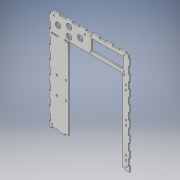
# Autodesk Inventor part: 10 voor plaat
Saved by Autodesk Inventor 2019 (Build 230136000, 136)
## iProperties
Created: 2021-01-22
Part Number: 10 voor plaat
Material: Generic
Document SubType Name: Sheet Metal
Designer: Stefan
Density: 1 g/cm^3
Sheet Metal Rule: Default_mm
Appearance: Default
Author: Stefan
Autodesk Inventor part; units mm, degrees
ref_plane "YZ Plane" through (0, 0, 0) normal (1, 0, 0) x (0, 1, 0)
ref_plane "XZ Plane" through (0, 0, 0) normal (0, 1, 0) x (-1, 0, 0)
ref_plane "XY Plane" through (0, 0, 0) normal (0, 0, 1) x (1, 0, 0)
sketch "Sketch1" plane through (0, 0, 0) normal (0, 0, 1) x (1, 0, 0)
  line L0 (-90.5, -90.5) -> (90.5, -90.5)
  line L1 (90.5, -90.5) -> (90.5, 90.5)
  line L2 (90.5, 90.5) -> (-90.5, 90.5)
  line L3 (-90.5, 90.5) -> (-90.5, -90.5)
  line L4 (-90.5, -90.5) -> (90.5, 90.5) construction
  line L5 (90.5, -90.5) -> (-90.5, 90.5) construction
  point P0 (0, 0)
  dimension "d0" = 181
  dimension "d1" = 181
  constraints: 12 end point, 2 midpoint, 2 parallel, 1 horizontal, 1 perpendicular
  measures "d0" distance of L2.end L1.end
  measures "d1" distance of L1.end L0.end
extrude "Extrusion1" add sketch "Sketch1" along normal blind 3
sketch "Sketch2" plane through (0, 0, 3) normal (0, 0, 1) x (1, 0, 0)
  line L0 (90.5, 90.5) -> (-90.5, 90.5) projected
  line L1 (-90.5, 90.5) -> (-85, 90.5)
  line L2 (-85, 90.5) -> (-85, 93.5)
  line L3 (-85, 93.5) -> (-90.5, 93.5)
  line L4 (-90.5, 93.5) -> (-90.5, 90.5)
  line L5 (80, 90.5) -> (85.5, 90.5)
  line L6 (85.5, 90.5) -> (85.5, 93.5)
  line L7 (85.5, 93.5) -> (80, 93.5)
  line L8 (80, 93.5) -> (80, 90.5)
  line L9 (-90.5, -93.5) -> (-85, -93.5)
  line L10 (-85, -93.5) -> (-85, -90.5)
  line L11 (-85, -90.5) -> (-90.5, -90.5)
  line L12 (-90.5, -90.5) -> (-90.5, -93.5)
  line L13 (80, -93.5) -> (85.5, -93.5)
  line L14 (85.5, -93.5) -> (85.5, -90.5)
  line L15 (85.5, -90.5) -> (80, -90.5)
  line L16 (80, -90.5) -> (80, -93.5)
  line L17 (-70, 90.5) -> (-55, 90.5)
  line L18 (-55, 90.5) -> (-55, 93.5)
  line L19 (-55, 93.5) -> (-70, 93.5)
  line L20 (-70, 93.5) -> (-70, 90.5)
  line L21 (-25, 90.5) -> (-25, 93.5)
  line L22 (-40, 90.5) -> (-25, 90.5)
  line L23 (-25, 93.5) -> (-40, 93.5)
  line L24 (-40, 93.5) -> (-40, 90.5)
  line L25 (5, 90.5) -> (5, 93.5)
  line L26 (-10, 90.5) -> (5, 90.5)
  line L27 (5, 93.5) -> (-10, 93.5)
  line L28 (-10, 93.5) -> (-10, 90.5)
  line L29 (35, 90.5) -> (35, 93.5)
  line L30 (20, 90.5) -> (35, 90.5)
  line L31 (35, 93.5) -> (20, 93.5)
  line L32 (20, 93.5) -> (20, 90.5)
  line L33 (65, 90.5) -> (65, 93.5)
  line L34 (50, 90.5) -> (65, 90.5)
  line L35 (65, 93.5) -> (50, 93.5)
  line L36 (50, 93.5) -> (50, 90.5)
  line L37 (-55, -93.5) -> (-55, -90.5)
  line L38 (-70, -93.5) -> (-55, -93.5)
  line L39 (-55, -90.5) -> (-70, -90.5)
  line L40 (-70, -90.5) -> (-70, -93.5)
  line L41 (-25, -93.5) -> (-25, -90.5)
  line L42 (-40, -93.5) -> (-25, -93.5)
  line L43 (-25, -90.5) -> (-40, -90.5)
  line L44 (-40, -90.5) -> (-40, -93.5)
  line L45 (5, -93.5) -> (5, -90.5)
  line L46 (-10, -93.5) -> (5, -93.5)
  line L47 (5, -90.5) -> (-10, -90.5)
  line L48 (-10, -90.5) -> (-10, -93.5)
  line L49 (35, -93.5) -> (35, -90.5)
  line L50 (20, -93.5) -> (35, -93.5)
  line L51 (35, -90.5) -> (20, -90.5)
  line L52 (20, -90.5) -> (20, -93.5)
  line L53 (65, -93.5) -> (65, -90.5)
  line L54 (50, -93.5) -> (65, -93.5)
  line L55 (65, -90.5) -> (50, -90.5)
  line L56 (50, -90.5) -> (50, -93.5)
  point P0 (0, 0)
  dimension "d4" = 5.5
  dimension "d5" = 3
  dimension "d8" = 170.5
  dimension "d11" = 184
  dimension "d14" = 15
  dimension "d15" = 3
  dimension "d16" = 15
  dimension "d19" = 30
  dimension "d22" = 184
  constraints: 112 end point, 4 horizontal, 4 parallel, 3 collinear, 2 perpendicular, 2 vertical, 1 point on line, 93 other
  measures "d4" distance of L3.end L2.end
  measures "d5" distance of L2.end L1.end
  measures "d8" distance of L2.end L6.end
  measures "d11" distance of L2.end L10.end
  measures "d14" distance of L19.end L18.end
  measures "d15" distance of L18.end L17.end
  measures "d16" distance between parallel lines of L20 L2
  measures "d19" distance of L17.end L21.start
  measures "d22" distance of L17.end L37.start
extrude "Extrusion2" add sketch "Sketch2" against normal blind 3
sketch "Sketch3" plane through (0, 0, 3) normal (0, 0, 1) x (1, 0, 0)
  line L0 (-90.5, 93.5) -> (-90.5, -93.5) projected
  line L1 (-90.5, 82.5) -> (-87.5, 82.5)
  line L2 (-87.5, 82.5) -> (-87.5, 67.5)
  line L3 (-87.5, 67.5) -> (-90.5, 67.5)
  line L4 (-90.5, 67.5) -> (-90.5, 82.5)
  line L5 (-85, 93.5) -> (-90.5, 93.5) projected
  line L6 (-90.5, 52.5) -> (-87.5, 52.5)
  line L7 (-87.5, 52.5) -> (-87.5, 37.5)
  line L8 (-87.5, 37.5) -> (-90.5, 37.5)
  line L9 (-90.5, 37.5) -> (-90.5, 52.5)
  line L10 (-90.5, 22.5) -> (-87.5, 22.5)
  line L11 (-87.5, 22.5) -> (-87.5, 7.5)
  line L12 (-87.5, 7.5) -> (-90.5, 7.5)
  line L13 (-90.5, 7.5) -> (-90.5, 22.5)
  line L14 (-90.5, -7.5) -> (-87.5, -7.5)
  line L15 (-87.5, -7.5) -> (-87.5, -22.5)
  line L16 (-87.5, -22.5) -> (-90.5, -22.5)
  line L17 (-90.5, -22.5) -> (-90.5, -7.5)
  line L18 (-90.5, -37.5) -> (-87.5, -37.5)
  line L19 (-87.5, -37.5) -> (-87.5, -52.5)
  line L20 (-87.5, -52.5) -> (-90.5, -52.5)
  line L21 (-90.5, -52.5) -> (-90.5, -37.5)
  line L22 (-90.5, -67.5) -> (-87.5, -67.5)
  line L23 (-87.5, -67.5) -> (-87.5, -82.5)
  line L24 (-87.5, -82.5) -> (-90.5, -82.5)
  line L25 (-90.5, -82.5) -> (-90.5, -67.5)
  line L26 (87.5, 82.5) -> (90.5, 82.5)
  line L27 (90.5, 82.5) -> (90.5, 67.5)
  line L28 (90.5, 67.5) -> (87.5, 67.5)
  line L29 (87.5, 67.5) -> (87.5, 82.5)
  line L30 (87.5, 52.5) -> (90.5, 52.5)
  line L31 (90.5, 52.5) -> (90.5, 37.5)
  line L32 (90.5, 37.5) -> (87.5, 37.5)
  line L33 (87.5, 37.5) -> (87.5, 52.5)
  line L34 (87.5, 22.5) -> (90.5, 22.5)
  line L35 (90.5, 22.5) -> (90.5, 7.5)
  line L36 (90.5, 7.5) -> (87.5, 7.5)
  line L37 (87.5, 7.5) -> (87.5, 22.5)
  line L38 (87.5, -7.5) -> (90.5, -7.5)
  line L39 (90.5, -7.5) -> (90.5, -22.5)
  line L40 (90.5, -22.5) -> (87.5, -22.5)
  line L41 (87.5, -22.5) -> (87.5, -7.5)
  line L42 (87.5, -37.5) -> (90.5, -37.5)
  line L43 (90.5, -37.5) -> (90.5, -52.5)
  line L44 (90.5, -52.5) -> (87.5, -52.5)
  line L45 (87.5, -52.5) -> (87.5, -37.5)
  line L46 (87.5, -67.5) -> (90.5, -67.5)
  line L47 (90.5, -67.5) -> (90.5, -82.5)
  line L48 (90.5, -82.5) -> (87.5, -82.5)
  line L49 (87.5, -82.5) -> (87.5, -67.5)
  point P0 (0, 0)
  dimension "d27" = 3
  dimension "d28" = 15
  dimension "d29" = 11
  dimension "d32" = 30
  dimension "d35" = 178
  constraints: 96 end point, 2 horizontal, 2 parallel, 1 perpendicular, 1 point on line, 1 vertical, 88 other
  measures "d27" distance of L2.end L3.end
  measures "d28" distance of L1.end L2.end
  measures "d29" distance between parallel lines of L5 L1
  measures "d32" distance of L1.start L6.start
  measures "d35" distance of L1.start L26.start
extrude "Extrusion3" cut sketch "Sketch3" against normal blind 3
sketch "Sketch4" plane through (0, 0, 3) normal (0, 0, 1) x (1, 0, 0)
  line L0 (80, 93.5) -> (85.5, 93.5) projected
  line L1 (90.5, 90.5) -> (85.5, 90.5) projected
  line L2 (85.5, 93.5) -> (90.5, 93.5)
  line L3 (90.5, 93.5) -> (90.5, 90.5)
  line L4 (90.5, 90.5) -> (85.5, 90.5)
  line L5 (85.5, 90.5) -> (85.5, 93.5)
  line L6 (85.5, -90.5) -> (90.5, -90.5) projected
  line L7 (85.5, -90.5) -> (90.5, -90.5)
  line L8 (90.5, -90.5) -> (90.5, -93.5)
  line L9 (90.5, -93.5) -> (85.5, -93.5)
  line L10 (85.5, -93.5) -> (85.5, -90.5)
  point P0 (0, 0)
  dimension "d40" = 184
  constraints: 16 end point, 4 parallel, 2 horizontal, 2 perpendicular, 1 point on line
  measures "d40" distance between parallel lines of L1 L9
extrude "Extrusion4" add sketch "Sketch4" against normal blind 3
sketch "Sketch5" plane through (0, 0, 0) normal (0, 0, -1) x (-1, 0, 0)
  line L0 (-75, 93.5) -> (47.5, 93.5)
  line L1 (47.5, 93.5) -> (47.5, -93.5)
  line L2 (47.5, -93.5) -> (-75, -93.5)
  line L3 (-75, -93.5) -> (-75, 93.5)
  line L4 (-90.5, 22.5) -> (-90.5, 37.5) projected
  line L5 (90.5, 22.5) -> (90.5, 37.5) projected
  point P0 (0, 0)
  dimension "d43" = 187
  dimension "d44" = 15.5
  dimension "d45" = 43
  dimension "d46" = 93.5
  constraints: 8 end point, 2 parallel, 1 horizontal, 1 perpendicular
  measures "d43" distance of L0.end L1.end
  measures "d44" distance between parallel lines of L3 L4
  measures "d45" distance between parallel lines of L5 L1
  measures "d46" distance from line of point (0, 0) L0
extrude "Extrusion5" cut sketch "Sketch5" against normal blind 10
sketch "Sketch6" plane through (0, 0, 0) normal (0, 0, -1) x (-1, 0, 0)
  line L0 (-87.5, 82.5) -> (-90.5, 82.5)
  circle A0 centre (-83, 73.5) radius 2
  circle A1 centre (-83, 63.5) radius 2
  line L1 (-87.5, 82.5) -> (-87.5, 67.5)
  line L2 (-80, 93.5) -> (-90.5, 93.5)
  circle A2 centre (-83, -73.5) radius 2
  circle A3 centre (-83, -63.5) radius 2
  line L3 (-87.5, -67.5) -> (-87.5, -82.5)
  line L4 (-90.5, -93.5) -> (-80, -93.5)
  circle A4 centre (-83, 5) radius 2
  circle A5 centre (-83, -5) radius 2
  line L5 (-87.5, 22.5) -> (-87.5, 7.5)
  line L6 (-90.5, -7.5) -> (-87.5, -7.5)
  line L7 (52.75, -25) -> (72.95, -25) construction
  line L8 (72.95, -25) -> (72.95, 15) construction
  line L9 (72.95, 15) -> (52.75, 15) construction
  line L10 (52.75, 15) -> (52.75, -25) construction
  circle A6 centre (52.75, 15) radius 2
  circle A7 centre (72.95, 15) radius 2
  circle A8 centre (72.95, -25) radius 2
  circle A9 centre (52.75, -25) radius 2
  point P0 (0, 0)
  point P1 (0, 0)
  dimension "d49" = 4
  dimension "d50" = 4
  dimension "d51" = 10
  dimension "d52" = 4.5
  dimension "d53" = 0
  dimension "d54" = 20
  dimension "d55" = 4
  dimension "d56" = 4
  dimension "d57" = 10
  dimension "d58" = 4.5
  dimension "d59" = 4.5
  dimension "d60" = 20
  dimension "d61" = 4
  dimension "d62" = 4
  dimension "d63" = 0
  dimension "d64" = 10
  dimension "d65" = 4.5
  dimension "d66" = 2.5
  dimension "d67" = 20.2
  dimension "d68" = 40
  dimension "d69" = 72.95
  dimension "d70" = 15
  dimension "d71" = 4
  dimension "d72" = 4
  dimension "d73" = 4
  dimension "d74" = 4
  dimension "d75" = 90
  dimension "d76" = 90
  dimension "d77" = 160.45
  dimension "d78" = 78.5
  dimension "d79" = 67.5
  dimension "d80" = 22.5
  dimension "d81" = 108.5
  dimension "d82" = 72.95
  dimension "d83" = 15
  dimension "d84" = 87.5
  dimension "d85" = 87.5
  dimension "d86" = 152.95
  dimension "d87" = 152.95
  dimension "d88" = 52.5
  dimension "d89" = 7.5
  dimension "d90" = 7.5
  dimension "d91" = 160.45
  dimension "d92" = 82.5
  dimension "d93" = 97.5
  dimension "d94" = 163.45
  dimension "d95" = 163.45
  dimension "d96" = 163.45
  dimension "d97" = 163.45
  constraints: 22 end point, 10 centre point, 7 parallel, 4 coincident, 1 horizontal, 1 perpendicular
  measures "d49" diameter of A0
  measures "d50" diameter of A1
  measures "d51" distance of A0.centre A1.centre
  measures "d52" distance from line of L1 A0.centre
  measures "d53" horizontal distance of A0.centre A1.centre
  measures "d54" distance from line of L2 A0.centre
  measures "d55" diameter of A2
  measures "d56" diameter of A3
  measures "d57" distance of A3.centre A2.centre
  measures "d58" distance from line of A3.centre L3
  measures "d59" distance from line of L3 A2.centre
  measures "d60" distance from line of L4 A2.centre
  measures "d61" diameter of A4
  measures "d62" diameter of A5
  measures "d63" horizontal distance of A4.centre A5.centre
  measures "d64" distance of A4.centre A5.centre
  measures "d65" distance from line of L5 A5.centre
  measures "d66" distance from line of A5.centre L6
  measures "d67" distance of L9.end L8.end
  measures "d68" distance of L8.end L7.end
  measures "d69" distance from line of point (0, 0) L8
  measures "d70" distance from line of point (0, 0) L9
  measures "d71" diameter of A6
  measures "d72" diameter of A9
  measures "d73" diameter of A8
  measures "d74" diameter of A7
  measures "d75" angle of L1 L9
  measures "d76" angle of L3 L9
  measures "d77" distance between parallel lines of L5 L8
  measures "d78" distance between parallel lines of L2 L9
  measures "d79" distance between parallel lines of L0 L9
  measures "d80" distance between parallel lines of L6 L9
  measures "d81" distance between parallel lines of L4 L9
  measures "d82" distance from line of point (0, 0) L8
  measures "d83" distance from line of point (0, 0) L9
  measures "d84" distance from line of point (0, 0) L1
  measures "d85" distance from line of point (0, 0) L3
  measures "d86" distance from line of L2.start L8
  measures "d87" distance from line of L4.end L8
  measures "d88" distance from line of L1.end L9
  measures "d89" distance from line of L5.start L9
  measures "d90" distance from line of L5.end L9
  measures "d91" distance from line of L6.end L8
  measures "d92" distance from line of L3.start L9
  measures "d93" distance from line of L3.end L9
  measures "d94" distance from line of L2.end L8
  measures "d95" distance from line of L0.end L8
  measures "d96" distance from line of L6.start L8
  measures "d97" distance from line of L4.start L8
extrude "Extrusion6" cut sketch "Sketch6" against normal blind 10
sketch "Sketch8" plane through (0, 0, 0) normal (0, 0, -1) x (-1, 0, 0)
  line L0 (-90.5, 82.5) -> (-90.5, 93.5)
  line L1 (-90.5, 93.5) -> (90.5, 93.5)
  line L2 (90.5, 93.5) -> (90.5, 133.5)
  line L3 (90.5, 133.5) -> (-90.5, 133.5)
  line L4 (-90.5, 133.5) -> (-90.5, 93.5)
  line L5 (-76.15, 101.2) -> (-4.85, 101.2)
  line L6 (-4.85, 101.2) -> (-4.85, 125.8)
  line L7 (-4.85, 125.8) -> (-76.15, 125.8)
  line L8 (-76.15, 125.8) -> (-76.15, 101.2)
  line L9 (-76.15, 101.2) -> (-4.85, 125.8) construction
  line L10 (-4.85, 101.2) -> (-76.15, 125.8) construction
  line L11 (-78.025, 98) -> (-2.975, 98) construction
  line L12 (-2.975, 98) -> (-2.975, 129) construction
  line L13 (-2.975, 129) -> (-78.025, 129) construction
  line L14 (-78.025, 129) -> (-78.025, 98) construction
  line L15 (-78.025, 98) -> (-2.975, 129) construction
  line L16 (-2.975, 98) -> (-78.025, 129) construction
  circle A0 centre (-2.975, 129) radius 1.5
  circle A1 centre (-2.975, 98) radius 1.5
  circle A2 centre (-78.025, 98) radius 1.5
  circle A3 centre (-78.025, 129) radius 1.5
  circle A4 centre (45.25, 103.75) radius 6.15
  circle A5 centre (45.25, 103.75) radius 8.25 construction
  circle A6 centre (70.25, 113.5) radius 6.15
  circle A7 centre (70.25, 113.5) radius 8.25 construction
  circle A8 centre (45.25, 123.25) radius 6.15
  circle A9 centre (45.25, 123.25) radius 8.25 construction
  circle A10 centre (20.25, 113.5) radius 6.15
  circle A11 centre (20.25, 113.5) radius 8.25 construction
  point P0 (0, 0)
  point P1 (0, 0)
  point P2 (-40.5, 113.5)
  dimension "d150" = 181
  dimension "d151" = 40
  dimension "d152" = 71.3
  dimension "d153" = 24.6
  dimension "d154" = 31
  dimension "d155" = 75.05
  dimension "d156" = 3
  dimension "d157" = 3
  dimension "d158" = 3
  dimension "d159" = 3
  dimension "d160" = 20
  dimension "d161" = 50
  dimension "d162" = 12.3
  dimension "d163" = 16.5
  dimension "d164" = 12.3
  dimension "d165" = 16.5
  dimension "d166" = 12.3
  dimension "d167" = 16.5
  dimension "d168" = 12.3
  dimension "d169" = 16.5
  dimension "d170" = 45.25
  dimension "d171" = 45.25
  dimension "d172" = 2
  dimension "d173" = 2
  dimension "d174" = 20
  dimension "d175" = 20
  dimension "d176" = 90.5
  dimension "d177" = 25
  dimension "d178" = 25
  dimension "d179" = 90
  dimension "d180" = 90.5
  dimension "d181" = 133.5
  dimension "d182" = 20.25
  dimension "d183" = 133.5
  dimension "d184" = 51
  constraints: 34 end point, 12 centre point, 8 coincident, 6 parallel, 4 midpoint, 3 horizontal, 3 perpendicular
  measures "d150" distance of L4.start L3.start
  measures "d151" distance of L3.start L1.end
  measures "d152" distance of L8.start L6.end
  measures "d153" distance of L6.end L6.start
  measures "d154" distance of L12.end L12.start
  measures "d155" distance of L12.end L14.start
  measures "d156" diameter of A0
  measures "d157" diameter of A1
  measures "d158" diameter of A2
  measures "d159" diameter of A3
  measures "d160" distance from line of L3 point (-40.5, 113.5)
  measures "d161" distance from line of point (-40.5, 113.5) L4
  measures "d162" diameter of A4
  measures "d163" diameter of A5
  measures "d164" diameter of A6
  measures "d165" diameter of A7
  measures "d166" diameter of A8
  measures "d167" diameter of A9
  measures "d168" diameter of A10
  measures "d169" diameter of A11
  measures "d170" horizontal distance of A9.centre point (0, 0)
  measures "d171" horizontal distance of A4.centre point (0, 0)
  measures "d172" distance edge to line of A9 L3
  measures "d173" distance edge to line of A5 L1
  measures "d174" distance from line of A6.centre L3
  measures "d175" distance from line of L3 A11.centre
  measures "d176" horizontal distance of L1.end point (0, 0)
  measures "d177" horizontal distance of A8.centre A11.centre
  measures "d178" horizontal distance of A9.centre A6.centre
  measures "d179" angle of L0 L3
  measures "d180" distance from line of point (0, 0) L2
  measures "d181" distance from line of point (0, 0) L3
  measures "d182" distance from line of A6.centre L2
  measures "d183" distance from line of point (0, 0) L3
  measures "d184" distance from line of L0.start L3
extrude "Extrusion8" add sketch "Sketch8" against normal blind 3
sketch "Sketch9" plane through (0, 0, 0) normal (0, 0, -1) x (-1, 0, 0)
  line L0 (8.25, 102.222) -> (14.25, 102.222)
  line L1 (15.25, 102.222) -> (15.25, 94.222)
  line L2 (15.25, 94.222) -> (7.25, 94.222)
  line L3 (7.25, 94.222) -> (7.25, 102.222)
  line L4 (7.25, 102.222) -> (15.25, 94.222) construction
  line L5 (15.25, 102.222) -> (7.25, 94.222) construction
  arc A0 (15.25, 102.222) -> (7.25, 102.222) centre (11.25, 102.222) ccw
  arc A1 (14.25, 102.222) -> (8.25, 102.222) centre (11.25, 102.222) ccw
  arc A2 (11.75, 97.356) -> (10.75, 97.356) centre (11.25, 98.222) ccw
  line L6 (10.75, 95.722) -> (11.75, 95.722)
  line L7 (10.75, 95.722) -> (11.75, 98.722) construction
  line L8 (11.75, 95.722) -> (10.75, 98.722) construction
  line L9 (10.75, 97.356) -> (10.75, 95.722)
  line L10 (11.75, 95.722) -> (11.75, 97.356)
  line L11 (55, 93.5) -> (-80, 93.5) projected
  circle A3 centre (20.25, 113.5) radius 6.15 projected
  circle A4 centre (20.25, 113.5) radius 8 construction
  point P0 (0, 0)
  dimension "d187" = 8
  dimension "d188" = 8
  dimension "d189" = 1
  dimension "d190" = 2
  dimension "d191" = 1
  dimension "d192" = 3
  dimension "d193" = 0.722
  dimension "d194" = 16
  dimension "d195" = 9
  dimension "d196" = 71.565
  dimension "d197" = 108.435
  dimension "d198" = 8.722
  dimension "d199" = 2.222
  dimension "d200" = 3.5
  dimension "d201" = 4.5
  constraints: 22 end point, 6 point on circle, 4 centre point, 3 parallel, 2 coincident, 2 horizontal, 2 midpoint, 2 perpendicular, 2 tangent
  measures "d187" distance of L1.end L2.end
  measures "d188" distance of L1.start L1.end
  measures "d189" radial gap between concentric circles of A0 A1
  measures "d190" diameter of A2
  measures "d191" distance of L8.end L7.end
  measures "d192" distance of L7.end L6.end
  measures "d193" distance between parallel lines of L11 L2
  measures "d194" diameter of A4
  measures "d195" horizontal distance of A4.centre point (11.25, 98.222)
  measures "d196" angle of L8 L11
  measures "d197" angle of L7 L11
  measures "d198" distance between parallel lines of L0 L11
  measures "d199" distance between parallel lines of L6 L11
  measures "d200" distance between parallel lines of L10 L1
  measures "d201" distance between parallel lines of L9 L1
extrude "Extrusion9" add sketch "Sketch9" along normal blind 0.2 contours L1 L2 L3 A0
sketch "Sketch10" plane through (0, 0, 0) normal (0, 0, -1) x (-1, 0, 0)
  circle A0 centre (45.25, 123.25) radius 6.15 construction
  circle A1 centre (45.25, 103.75) radius 6.15 construction
  circle A2 centre (45.25, 103.75) radius 8 construction
  circle A3 centre (70.25, 113.5) radius 6.15 construction
  circle A4 centre (70.25, 113.5) radius 8 construction
  line L0 (32.25, 123.25) -> (32.25, 131.6682) construction
  line L1 (32.25, 103.75) -> (32.25, 95.75) construction
  line L2 (32.25, 131.6682) -> (35.8952, 125.3545)
  line L3 (35.8952, 125.3545) -> (28.6048, 125.3545)
  line L4 (28.6048, 125.3545) -> (32.25, 131.6682)
  line L5 (32.25, 95.75) -> (28.7859, 101.75)
  line L6 (28.7859, 101.75) -> (35.7141, 101.75)
  line L7 (35.7141, 101.75) -> (32.25, 95.75)
  line L8 (70.25, 113.5) -> (58.25, 113.5) construction
  line L9 (53.0987, 113.4997) -> (54.5129, 114.9139)
  line L10 (54.5129, 114.9139) -> (55.9271, 113.4997)
  line L11 (53.0987, 113.4997) -> (55.0987, 113.4997) construction
  line L12 (55.9271, 113.4997) -> (60.1698, 117.7424)
  line L13 (60.1698, 117.7424) -> (61.584, 116.3281)
  line L14 (61.584, 116.3281) -> (55.9271, 110.6713)
  line L15 (53.0987, 113.4997) -> (55.9271, 110.6713)
  line L16 (32.25, 123.25) -> (45.25, 123.25) construction
  line L17 (32.25, 103.75) -> (45.25, 103.75) construction
  circle A5 centre (45.25, 123.25) radius 8 construction
  point P0 (0, 0)
  point P1 (32.25, 127.4591)
  point P2 (32.25, 99.75)
  dimension "d205" = 16
  dimension "d206" = 16
  dimension "d207" = 13
  dimension "d208" = 13
  dimension "d211" = 12
  dimension "d212" = 2
  dimension "d213" = 45
  dimension "d217" = 6
  dimension "d218" = 2
  dimension "d219" = 4.128
  dimension "d223" = 0.0003
  dimension "d224" = 4
  dimension "d259" = 16
  dimension "d260" = 11.8545
  dimension "d261" = 11.75
  constraints: 36 end point, 6 parallel, 4 horizontal, 3 centre point, 3 coincident, 2 midpoint, 1 equal length, 1 perpendicular, 14 other
  measures "d205" diameter of A2
  measures "d206" diameter of A4
  measures "d207" distance of L16.end L0.start
  measures "d208" distance of L17.end L1.start
  measures "d211" distance of L8.start L8.end
  measures "d212" distance of L9.start L9.end
  measures "d213" angle of L11 L9
  measures "d217" distance between parallel lines of L13 L10
  measures "d218" distance between parallel lines of L14 L12
  measures "d219" distance from line of L8.start L13
  measures "d223" distance between parallel lines of L8 L11
  measures "d224" distance between parallel lines of L14 L9
  measures "d259" diameter of A5
  measures "d260" distance between parallel lines of L3 L8
  measures "d261" distance between parallel lines of L8 L6
extrude "Extrusion10" add sketch "Sketch10" along normal blind 0.2
fillet "Fillet1" radius 0.75 5 edges at (-61.584, 116.3281, -0.1) (-60.1698, 117.7424, -0.1) (-54.5129, 114.9139, -0.1) (-53.0987, 113.4997, -0.1) (-55.9271, 110.6713, -0.1)
sketch "Sketch11" plane through (0, 0, 0) normal (0, 0, -1) x (-1, 0, 0)
  line L0 (-90.5, 82.5) -> (-90.5, 97.5) construction
  line L1 (-90.5, 97.5) -> (-87.5, 97.5)
  line L2 (-87.5, 97.5) -> (-87.5, 112.5)
  line L3 (-87.5, 112.5) -> (-90.5, 112.5)
  line L4 (-90.5, 112.5) -> (-90.5, 97.5)
  line L5 (-90.5, 112.5) -> (-90.5, 127.5) construction
  line L6 (-90.5, 127.5) -> (-87.5, 127.5)
  line L7 (-87.5, 127.5) -> (-87.5, 133.5)
  line L8 (-90.5, 133.5) -> (-90.5, 127.5)
  line L9 (90.5, 82.5) -> (87.5, 82.5) construction
  line L10 (90.5, 82.5) -> (90.5, 97.5) construction
  line L11 (90.5, 97.5) -> (87.5, 97.5)
  line L12 (87.5, 97.5) -> (87.5, 112.5)
  line L13 (87.5, 112.5) -> (90.5, 112.5)
  line L14 (90.5, 112.5) -> (90.5, 97.5)
  line L15 (90.5, 112.5) -> (90.5, 127.5) construction
  line L16 (90.5, 127.5) -> (87.5, 127.5)
  line L17 (87.5, 127.5) -> (87.5, 133.5)
  line L18 (87.5, 133.5) -> (90.5, 133.5)
  line L19 (90.5, 133.5) -> (90.5, 127.5)
  line L20 (-90.5, 133.5) -> (90.5, 133.5) construction
  line L21 (-90.5, 133.5) -> (-87.5, 133.5)
  point P0 (0, 0)
  dimension "d225" = 15
  dimension "d226" = 3
  dimension "d227" = 15
  dimension "d228" = 15
  dimension "d229" = 15
  dimension "d230" = 3
  dimension "d231" = 15
  dimension "d232" = 15
  dimension "d233" = 90
  dimension "d234" = 90
  dimension "d235" = 3
  dimension "d236" = 178
  constraints: 40 end point, 7 parallel, 4 horizontal, 4 perpendicular, 1 collinear
  measures "d225" distance of L0.start L0.end
  measures "d226" distance of L3.end L2.end
  measures "d227" distance of L2.end L1.end
  measures "d228" distance of L3.end L5.end
  measures "d229" distance of L9.start L10.end
  measures "d230" distance of L12.end L13.end
  measures "d231" distance of L11.end L12.end
  measures "d232" distance of L13.end L15.end
  measures "d233" angle of L9 L15
  measures "d234" angle of L9 L5
  measures "d235" distance between parallel lines of L17 L19
  measures "d236" distance between parallel lines of L19 L7
extrude "Extrusion11" cut sketch "Sketch11" against normal blind 3
sketch "Sketch12" plane through (0, 0, 0) normal (0, 0, -1) x (-1, 0, 0)
  line L0 (-87.5, 133.5) -> (87.5, 133.5) projected
  line L1 (-82.5, 133.5) -> (-67.5, 133.5)
  line L2 (-67.5, 133.5) -> (-67.5, 136.5)
  line L3 (-67.5, 136.5) -> (-82.5, 136.5)
  line L4 (-82.5, 136.5) -> (-82.5, 133.5)
  line L5 (-90.5, 112.5) -> (-90.5, 127.5) projected
  line L6 (-52.5, 133.5) -> (-37.5, 133.5)
  line L7 (-37.5, 133.5) -> (-37.5, 136.5)
  line L8 (-37.5, 136.5) -> (-52.5, 136.5)
  line L9 (-52.5, 136.5) -> (-52.5, 133.5)
  line L10 (-22.5, 133.5) -> (-7.5, 133.5)
  line L11 (-7.5, 133.5) -> (-7.5, 136.5)
  line L12 (-7.5, 136.5) -> (-22.5, 136.5)
  line L13 (-22.5, 136.5) -> (-22.5, 133.5)
  line L14 (7.5, 133.5) -> (22.5, 133.5)
  line L15 (22.5, 133.5) -> (22.5, 136.5)
  line L16 (22.5, 136.5) -> (7.5, 136.5)
  line L17 (7.5, 136.5) -> (7.5, 133.5)
  line L18 (37.5, 133.5) -> (52.5, 133.5)
  line L19 (52.5, 133.5) -> (52.5, 136.5)
  line L20 (52.5, 136.5) -> (37.5, 136.5)
  line L21 (37.5, 136.5) -> (37.5, 133.5)
  line L22 (67.5, 133.5) -> (82.5, 133.5)
  line L23 (82.5, 133.5) -> (82.5, 136.5)
  line L24 (82.5, 136.5) -> (67.5, 136.5)
  line L25 (67.5, 136.5) -> (67.5, 133.5)
  point P0 (0, 0)
  dimension "d239" = 15
  dimension "d240" = 3
  dimension "d241" = 8
  dimension "d244" = 30
  constraints: 48 end point, 2 horizontal, 2 parallel, 1 perpendicular, 1 point on line, 40 other
  measures "d239" distance of L3.end L2.end
  measures "d240" distance of L2.end L1.end
  measures "d241" distance between parallel lines of L5 L4
  measures "d244" distance of L1.start L6.start
extrude "Extrusion12" add sketch "Sketch12" against normal blind 3
sketch "Sketch13" plane through (0, 0, 3) normal (0, 0, 1) x (1, 0, 0)
  circle A0 centre (-84, -86) radius 1.5
  circle A1 centre (84, -86) radius 1.5
  line L0 (-90.5, -82.5) -> (-90.5, -93.5) projected
  line L1 (-85, -93.5) -> (-90.5, -93.5) projected
  line L2 (90.5, -93.5) -> (80, -93.5) projected
  line L3 (90.5, -82.5) -> (90.5, -93.5) projected
  point P0 (0, 0)
  dimension "d251" = 3
  dimension "d252" = 3
  dimension "d253" = 6.5
  dimension "d254" = 7.5
  dimension "d255" = 7.5
  dimension "d256" = 6.5
  constraints: 2 centre point
  measures "d251" diameter of A0
  measures "d252" diameter of A1
  measures "d253" distance from line of L0 A0.centre
  measures "d254" distance from line of L1 A0.centre
  measures "d255" distance from line of L2 A1.centre
  measures "d256" distance from line of L3 A1.centre
extrude "Extrusion13" cut sketch "Sketch13" against normal blind 10
sketch "Sketch14" plane through (0, 0, 0) normal (0, 0, -1) x (-1, 0, 0)
  circle A0 centre (9.5, 125.5) radius 2
  line L0 (-7.5, 133.5) -> (7.5, 133.5) projected
  line L1 (7.5, 136.5) -> (7.5, 133.5) projected
  circle A1 centre (79.5, 128.5) radius 2
  line L2 (87.5, 127.5) -> (87.5, 133.5) projected
  line L3 (82.5, 133.5) -> (87.5, 133.5) projected
  point P0 (0, 0)
  dimension "d262" = 4
  dimension "d263" = 8
  dimension "d264" = 2
  dimension "d267" = 4
  dimension "d268" = 8
  dimension "d269" = 5
  constraints: 2 centre point
  measures "d262" diameter of A0
  measures "d263" distance from line of A0.centre L0
  measures "d264" distance from line of A0.centre L1
  measures "d267" diameter of A1
  measures "d268" distance from line of L2 A1.centre
  measures "d269" distance from line of A1.centre L3
extrude "Extrusion14" cut sketch "Sketch14" against normal blind 10
equation "\"d72\" = d71"
equation "\"d73\" = d71"
equation "\"d74\" = d71"
equation "\"BendRadius\" = Thickness"
equation "\"BendReliefWidth\" = Thickness"
equation "\"BendReliefDepth\" = 0.5 * Thickness"
equation "\"CornerReliefSize\" = 4 * Thickness"
equation "\"MinimumRemnant\" = 2 * Thickness"
equation "\"TransitionRadius\" = BendRadius"
equation "\"JacobiRadiusSize\" = BendRadius"
equation "\"GapSize\" = Thickness"
equation "\"Thickness\" = 0.5"
body "Solid1"
